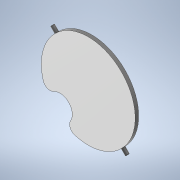
# Autodesk Inventor part: coin
Saved by Autodesk Inventor 2022 (Build 260153000, 153)
## iProperties
Created: 2022-02-07
Part Number: coin
Material: ABS Plastic
Document SubType Name: Modeling
Designer: joshw
Density: 1.06 g/cm^3
Appearance: Smooth - White
Author: joshw
Autodesk Inventor part; units mm, degrees
ref_plane "YZ Plane" through (0, 0, 0) normal (1, 0, 0) x (0, 1, 0)
ref_plane "XZ Plane" through (0, 0, 0) normal (0, 1, 0) x (-1, 0, 0)
sketch "Sketch1" plane through (0, 0, 0) normal (0, 0, 1) x (1, 0, 0)
  circle A0 centre (-4, -4) radius 0.9814 construction
  circle A1 centre (4, 4) radius 0.9814 construction
  line L0 (-7, -7) -> (7, -7) construction
  line L1 (-7, 7) -> (-7, -7) construction
  line L2 (7, 7) -> (-7, 7) construction
  line L3 (7, -7) -> (7, 7) construction
  line L4 (0, -7) -> (0, 7)
  line L5 (-7, 0) -> (7, 0)
  arc A2 (-1.9207, -6.3543) -> (-6.3543, -1.9207) centre (0, 0) ccw
  arc A3 (-2.4927, -4.8891) -> (-4.8891, -2.4927) centre (-4, -4) ccw
  arc A4 (-2.4927, -4.8891) -> (-1.9207, -6.3543) centre (-1.6313, -5.3971) ccw
  arc A5 (-6.3543, -1.9207) -> (-4.8891, -2.4927) centre (-5.3971, -1.6313) ccw
  point P0 (0, 0)
  dimension "d0" = 3
  dimension "d1" = 3
  dimension "d2" = 3
  dimension "d3" = 3
  dimension "d4" = 3.5
  dimension "d5" = 1
  constraints: 12 end point, 8 point on circle, 6 centre point, 6 tangent, 5 midpoint, 1 coincident, 1 equal radius
  measures "d0" distance from line of L0 A0.centre
  measures "d1" distance from line of L1 A0.centre
  measures "d2" distance from line of L2 A1.centre
  measures "d3" distance from line of L3 A1.centre
  measures "d4" diameter of A3
  measures "d5" radius of A4
extrude "Extrusion1" add sketch "Sketch1" along normal mid plane 0.5
sketch "Sketch4" plane through (0, 0, 0) normal (0, 0, 1) x (1, 0, 0)
  line L0 (5.3033, -5.3033) -> (-5.3033, 5.3033)
  line L1 (0, 0) -> (0, 0.8225) construction
  dimension "d9" = 45
  dimension "d11" = 7.5
  dimension "d12" = 7.5
  constraints: 4 end point, 1 midpoint, 1 vertical
  measures "d9" angle of L1 L0
  measures "d11" distance of L0.start L1.start
  measures "d12" distance of L0.end L1.start
ref_plane "Work Plane1" through (5.3033, -5.3033, 0) normal (-0.7071068, 0.7071068, 0) x (-0.7071068, -0.7071068, 0)
sketch "Sketch5" plane through (5.3033, -5.3033, 0) normal (-0.7071068, 0.7071068, 0) x (-0.7071068, -0.7071068, 0)
  circle A0 centre (0, 0) radius 0.25
  point P0 (0, 0)
  dimension "d10" = 0.5
  constraints: 1 centre point, 1 coincident
  measures "d10" diameter of A0
sweep "Sweep1" add profiles "Sketch5" path "Sketch4"
fillet "Fillet1" radius 0.05 2 edges at (5.4801, -5.1265, 0) (-5.1265, 5.4801, 0)
body "Solid1"
